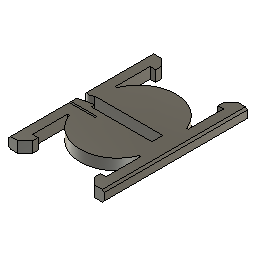
cable chain accessories v8 (Autodesk Fusion 360 design; units mm, degrees)
Autodesk Fusion 360 part; units mm, degrees
sketch "separator" plane through (0, 0, 0) normal (0, 0, 1) x (1, 0, 0)
  line L0 (0, 0) -> (57, 0)
  line L1 (57, 0) -> (57, 9)
  line L2 (57, 9) -> (0, 9)
  line L3 (0, 9) -> (0, 0)
  line L4 (0, 9) -> (57, 0) construction
  line L5 (41.5, 0) -> (15.5, 0) construction
  line L6 (15.5, 0) -> (15.5, 9)
  line L7 (15.5, 9) -> (41.5, 9) construction
  line L8 (41.5, 9) -> (41.5, 0)
  line L9 (41.5, 0) -> (15.5, 9) construction
  line L10 (15.5, 0) -> (41.5, 9) construction
  line L11 (12.5, 9) -> (12.5, 0)
  line L12 (44.5, 9) -> (44.5, 0)
  line L13 (16.5, 0) -> (16.5, 9)
  line L14 (40.5, 9) -> (40.5, 0)
  point P0 (28.5, 4.5)
  dimension "d1" = 57
  dimension "d2" = 9
  dimension "d3" = 26
  dimension "d4" = 9
  dimension "d5" = 3
  dimension "d6" = 3
  dimension "d7" = 1
  dimension "d8" = 1
  constraint horizontal L0
  constraint vertical L1
  constraint horizontal L2
  constraint vertical L3
  constraint coincident L0.start L3.end
  constraint horizontal L5
  constraint perpendicular L5 L6
  constraint parallel L5 L7
  constraint parallel L6 L8
  constraint coincident L9 P0
  constraint coincident L10 P0
  constraint midpoint L4 P0
  constraint coincident L2 L11.start
  constraint perpendicular L2 L11
  constraint coincident L2 L12.start
  constraint coincident L0 L12.end
  constraint perpendicular L0 L12
  measures "d1" distance of L0.start L0.end
  measures "d2" distance of L0.start L2.end
  measures "d3" distance of L6.end L7.end
  measures "d4" distance of L5.end L6.end
  measures "d5" distance of L6 L11
  measures "d6" distance of L8 L12
extrude "Extrude1" add sketch "separator" against normal blind 2 makes body 1
extrude "Extrude2" add sketch "separator" along normal blind 3.5 contours L0 L2 L6 L11 | L0 L2 L8 L12 bodies 1
extrude "Extrude3" add sketch "separator" along normal blind 1.5 from surface at 2 contours L0 L2 L6 L13 | L0 L2 L8 L14 bodies 1
fillet "Fillet1" radius 0.75 4 edges at (16.5, 4.5, 3.5) (16.5, 4.5, 2) (40.5, 4.5, 2) (40.5, 4.5, 3.5) on bodies 1
chamfer "Chamfer1" distance 1 angle 45 2 edges at (44.5, 4.5, 3.5) (12.5, 4.5, 3.5) on bodies 1
sketch "Sketch2" plane through (0, 0, 0) normal (0, 0, 1) x (1, 0, 0)
  line L0 (0, 0) -> (80, 0)
  line L1 (80, 0) -> (80, 39)
  line L2 (80, 39) -> (0, 39)
  line L3 (0, 39) -> (0, 0)
  line L4 (11, 39) -> (11, 0)
  line L5 (69, 39) -> (69, 0)
  line L6 (0, 6.5) -> (80, 6.5)
  line L7 (0, 39) -> (80, 0) construction
  line L8 (74.5, 11.5) -> (5.5, 11.5) construction
  line L9 (5.5, 11.5) -> (5.5, 27.5) construction
  line L10 (5.5, 27.5) -> (74.5, 27.5) construction
  line L11 (74.5, 27.5) -> (74.5, 11.5) construction
  line L12 (74.5, 11.5) -> (5.5, 27.5) construction
  line L13 (5.5, 11.5) -> (74.5, 27.5) construction
  circle A0 centre (5.5, 27.5) radius 2
  circle A1 centre (74.5, 27.5) radius 2
  circle A2 centre (5.5, 11.5) radius 2
  circle A3 centre (74.5, 11.5) radius 2
  arc A4 (13, 3) -> (22, 3) centre (17.5, 7.0625) ccw
  line L14 (22, 3) -> (22.6171, 6.5)
  line L15 (22, 3) -> (27, 3) construction
  line L16 (13, 3) -> (12.0622, 6.5)
  line L17 (13, 3) -> (16.8618, 3) construction
  line L18 (20.6035, 3.7181) -> (21.094, 6.5)
  arc A5 (14.3483, 3.7635) -> (20.6035, 3.7181) centre (17.5, 7.0625) ccw
  line L19 (14.3483, 3.7635) -> (13.6151, 6.5)
  arc A6 (24.5, 3) -> (33.5, 3) centre (29, 7.0625) ccw
  arc A7 (25.8483, 3.7635) -> (32.1035, 3.7181) centre (29, 7.0625) ccw
  line L20 (32.1035, 3.7181) -> (32.594, 6.5)
  line L21 (33.5, 3) -> (34.1171, 6.5)
  line L22 (25.8483, 3.7635) -> (25.1151, 6.5)
  line L23 (24.5, 3) -> (23.5622, 6.5)
  arc A8 (36, 3) -> (45, 3) centre (40.5, 7.0625) ccw
  arc A9 (37.3483, 3.7635) -> (43.6035, 3.7181) centre (40.5, 7.0625) ccw
  line L24 (43.6035, 3.7181) -> (44.094, 6.5)
  line L25 (45, 3) -> (45.6171, 6.5)
  line L26 (37.3483, 3.7635) -> (36.6151, 6.5)
  line L27 (36, 3) -> (35.0622, 6.5)
  arc A10 (47.5, 3) -> (56.5, 3) centre (52, 7.0625) ccw
  arc A11 (48.8483, 3.7635) -> (55.1035, 3.7181) centre (52, 7.0625) ccw
  line L28 (55.1035, 3.7181) -> (55.594, 6.5)
  line L29 (56.5, 3) -> (57.1171, 6.5)
  line L30 (48.8483, 3.7635) -> (48.1151, 6.5)
  line L31 (47.5, 3) -> (46.5622, 6.5)
  arc A12 (59, 3) -> (68, 3) centre (63.5, 7.0625) ccw
  arc A13 (60.3483, 3.7635) -> (66.6035, 3.7181) centre (63.5, 7.0625) ccw
  line L32 (66.6035, 3.7181) -> (67.094, 6.5)
  line L33 (68, 3) -> (68.6171, 6.5)
  line L34 (60.3483, 3.7635) -> (59.6151, 6.5)
  line L35 (59, 3) -> (58.0622, 6.5)
  point P0 (40, 19.5)
  dimension "d19" = 80
  dimension "d20" = 39
  dimension "d21" = 11
  dimension "d22" = 11
  dimension "d23" = 6.5
  dimension "d24" = 69
  dimension "d25" = 16
  dimension "d26" = 4
  dimension "d27" = 4
  dimension "d28" = 4
  dimension "d29" = 4
  dimension "d44" = 80
  dimension "d46" = 105
  dimension "d60" = 46
  dimension "d61" = 0
  constraint horizontal L0
  constraint vertical L1
  constraint horizontal L2
  constraint vertical L3
  constraint coincident L0.start L3.end
  constraint coincident L2 L4.start
  constraint coincident L0 L4.end
  constraint perpendicular L0 L4
  constraint coincident L2 L5.start
  constraint coincident L0 L5.end
  constraint perpendicular L0 L5
  constraint perpendicular L5 L6
  constraint horizontal L8
  constraint perpendicular L8 L9
  constraint parallel L8 L10
  constraint parallel L9 L11
  constraint coincident L12 P0
  constraint coincident L13 P0
  constraint midpoint L7 P0
  constraint coincident L9.end L10.start
  constraint coincident L10.end L11.start
  constraint coincident L8.end L9.start
  constraint coincident L8.start L11.end
  constraint coincident L3 L6.start
  constraint coincident L1 L6.end
  constraint horizontal L15
  constraint horizontal L17
  constraint coincident L6 L16.end
  constraint concentric A4 A5
  constraint coincident L6 L18.end
  constraint coincident L6 L14.end
  constraint coincident L6 L19.end
  measures "d19" distance of L0.start L0.end
  measures "d20" distance of L0.start L2.end
  measures "d21" distance of L3 L4
  measures "d22" distance of L1 L5
  measures "d23" distance of L0 L6
  measures "d24" distance of L9.end L10.end
  measures "d25" distance of L8.end L9.end
  measures "d26" diameter of A0
  measures "d27" diameter of A1
  measures "d28" diameter of A2
  measures "d29" diameter of A3
  measures "d44" angle of L14 L15
  measures "d46" angle of L16 L17
extrude "Extrude5" add sketch "Sketch2" along normal blind 40 separate body contours L0 L3 L4 L6 | L0 L4 L5 L6 A4 L14 L16 A6 L21 L23 A8 L25 L27 A10 L29 L31 A12 L33 L35 | L0 L1 L5 L6 | L6 A4 L14 L16 L18 A5 L19 | L6 A12 A13 L32 L33 L34 L35 | L6 L18 A5 L19 | L6 A13 L32 L34 | L6 A6 A7 L20 L21 L22 L23 | L6 A10 A11 L28 L29 L30 L31 | L6 A7 L20 L22 | L6 A11 L28 L30 | L6 A8 A9 L24 L25 L26 L27 | L6 A9 L24 L26 makes body 2
extrude "Extrude6" add sketch "Sketch2" along normal blind 25 contours L2 L3 L4 L6 | L1 L2 L5 L6 bodies 2
chamfer "Chamfer2" distance 15 angle 45 2 edges at (5.5, 39, 25) (74.5, 39, 25) on bodies 2
chamfer "Chamfer3" distance 5 angle 45 2 edges at (80, 3.25, 40) (0, 3.25, 40) on bodies 2
chamfer "Chamfer4" distance 1 angle 45 12 edges at (11, 15.25, 25) (11, 31.5, 17.5) (0, 31.5, 17.5) (0, 15.25, 25) (11, 39, 5) (0, 39, 5) (69, 39, 5) (80, 39, 5) (80, 31.5, 17.5) (69, 31.5, 17.5) (80, 15.25, 25) (69, 15.25, 25) on bodies 2
chamfer "Chamfer5" distance 1 angle 45 5 edges at (0, 6.5, 29.5) (2.5, 6.5, 37.5) (40, 6.5, 40) (77.5, 6.5, 37.5) (80, 6.5, 29.5) on bodies 2
extrude "Extrude10" cut sketch "Sketch2" along normal blind 3 from surface at 15 contours L6 A4 L14 L16 L18 A5 L19 | L6 A12 A13 L32 L33 L34 L35 | L6 A6 A7 L20 L21 L22 L23 | L6 A10 A11 L28 L29 L30 L31 | L6 A8 A9 L24 L25 L26 L27 bodies 2
extrude "Extrude11" cut sketch "Sketch2" along normal blind 3 from surface at 32 contours L6 A4 L14 L16 L18 A5 L19 | L6 A12 A13 L32 L33 L34 L35 | L6 A6 A7 L20 L21 L22 L23 | L6 A10 A11 L28 L29 L30 L31 | L6 A8 A9 L24 L25 L26 L27 bodies 2
chamfer "Chamfer6" distance 1 angle 45 5 edges at (80, 0, 17.5) (77.5, 0, 37.5) (40, 0, 40) (2.5, 0, 37.5) (0, 0, 17.5) on bodies 2
chamfer "Chamfer7" distance 1 angle 45 4 edges at (3.6353, 12.2232, 0) (3.6353, 28.2232, 0) (72.6353, 28.2232, 0) (72.6353, 12.2232, 0) on bodies 2
sketch "Sketch3" plane through (0, 0, 0) normal (0, 0, 1) x (1, 0, 0)
  line L0 (0, 0) -> (26, 0)
  line L1 (26, 0) -> (26, 39)
  line L2 (26, 39) -> (0, 39)
  line L3 (0, 39) -> (0, 0)
  line L4 (3, 35.5) -> (23, 35.5)
  line L5 (23, 35.5) -> (23, 32)
  line L6 (23, 32) -> (3, 32)
  line L7 (3, 32) -> (3, 35.5)
  line L8 (4.5, 39) -> (21.5, 39)
  line L9 (21.5, 39) -> (21.5, 35.5)
  line L10 (21.5, 35.5) -> (4.5, 35.5)
  line L11 (4.5, 35.5) -> (4.5, 39)
  line L12 (0, 19.5) -> (26, 19.5) construction
  line L13 (23, 7) -> (3, 7)
  line L14 (3, 7) -> (3, 3.5)
  line L15 (21.5, 3.5) -> (4.5, 3.5)
  line L16 (3, 3.5) -> (23, 3.5)
  line L17 (4.5, 3.5) -> (4.5, 0)
  line L18 (21.5, 0) -> (21.5, 3.5)
  line L19 (23, 3.5) -> (23, 7)
  line L20 (23, 7) -> (22.5, 7)
  line L21 (22.5, 7) -> (22.5, 13)
  line L22 (22.5, 13) -> (23, 13)
  line L23 (23, 13) -> (23, 7)
  line L24 (3, 7) -> (3.5, 7)
  line L25 (3.5, 7) -> (3.5, 13)
  line L26 (3.5, 13) -> (3, 13)
  line L27 (3, 13) -> (3, 7)
  line L28 (23, 32) -> (22.5, 32)
  line L29 (22.5, 32) -> (22.5, 26)
  line L30 (22.5, 26) -> (23, 26)
  line L31 (23, 26) -> (23, 32)
  line L32 (3, 32) -> (3.5, 32)
  line L33 (3.5, 32) -> (3.5, 26)
  line L34 (3.5, 26) -> (3, 26)
  line L35 (3, 26) -> (3, 32)
  arc A0 (22.5, 26) -> (3.5, 26) centre (13, 22.3563) ccw
  arc A1 (3.5, 13) -> (22.5, 13) centre (13, 16.6437) ccw
  dimension "d70" = 26
  dimension "d71" = 39
  dimension "d72" = 20
  dimension "d73" = 3.5
  dimension "d74" = 3
  dimension "d76" = 17
  dimension "d77" = 4.5
  dimension "d81" = 3.5
  dimension "d93" = 0.5
  dimension "d94" = 6
  dimension "d95" = 0.5
  dimension "d96" = 6
  dimension "d97" = 0.5
  dimension "d98" = 6
  dimension "d99" = 0.5
  dimension "d100" = 6
  constraint horizontal L0
  constraint vertical L1
  constraint horizontal L2
  constraint vertical L3
  constraint coincident L0.start L3.end
  constraint perpendicular L4 L5
  constraint parallel L4 L6
  constraint parallel L5 L7
  constraint perpendicular L1 L4
  constraint horizontal L8
  constraint vertical L9
  constraint horizontal L10
  constraint vertical L11
  constraint coincident L4 L9.end
  constraint coincident L2 L8.start
  constraint midpoint L3 L12.start
  constraint midpoint L1 L12.end
  constraint symmetric L4.start L12 L14.end
  constraint symmetric L4.end L12 L16.end
  constraint symmetric L5.end L12 L13.start
  constraint symmetric L6.end L12 L13.end
  constraint symmetric L8.start L12 L17.end
  constraint symmetric L8.end L12 L18.start
  constraint symmetric L9.end L12 L15.start
  constraint symmetric L10.end L12 L15.end
  constraint horizontal L20
  constraint vertical L21
  constraint horizontal L22
  constraint vertical L23
  constraint horizontal L24
  constraint vertical L25
  constraint horizontal L26
  constraint vertical L27
  constraint horizontal L28
  constraint vertical L29
  constraint horizontal L30
  constraint vertical L31
  constraint horizontal L32
  constraint vertical L33
  constraint horizontal L34
  constraint vertical L35
  constraint symmetric L12 L29.end L21.end
  constraint symmetric L12 L33.end L25.end
  constraint symmetric L12 A0 A1
  measures "d70" distance of L0.start L0.end
  measures "d71" distance of L0.start L2.end
  measures "d72" distance of L4.start L4.end
  measures "d73" distance of L4.start L6.end
  measures "d74" distance of L3 L7
  measures "d76" distance of L8.start L8.end
  measures "d77" distance of L3 L11
  measures "d81" distance of L2 L4
  measures "d93" distance of L13.start L20.end
  measures "d94" distance of L13.start L22.end
  measures "d95" distance of L13.end L24.end
  measures "d96" distance of L13.end L26.end
  measures "d97" distance of L5.end L28.end
  measures "d98" distance of L5.end L30.end
  measures "d99" distance of L6.end L32.end
  measures "d100" distance of L6.end L34.end
extrude "Extrude12" add sketch "Sketch3" along normal blind 3 separate body contours L0 L1 L2 L3 L4 L5 L6 L7 L9 L11 L13 L14 L16 L17 L18 L19 L22 L23 L26 L27 L30 L31 L34 L35 A0 A1 | L13 L24 L25 L26 L27 | L13 L20 L21 L22 L23 | L13 L25 A1 | L6 L32 L33 L34 L35 | L13 L21 A1 | L6 L28 L29 L30 L31 | L6 L33 A0 | L6 L29 A0 makes body 3
sketch "Sketch4" plane through (0, 0, 0) normal (0, 0, -1) x (1, 0, 0)
  line L0 (0, 0) -> (0, -39)
  line L1 (0, -39) -> (4.5, -39)
  line L2 (4.5, -39) -> (4.5, -35.5)
  line L3 (4.5, -35.5) -> (3, -35.5)
  line L4 (3, -35.5) -> (3, -32)
  line L5 (3, -32) -> (23, -32)
  line L6 (23, -32) -> (23, -35.5)
  line L7 (23, -35.5) -> (21.5, -35.5)
  line L8 (21.5, -35.5) -> (21.5, -39)
  line L9 (21.5, -39) -> (26, -39)
  line L10 (26, -39) -> (26, 0)
  line L11 (26, 0) -> (21.5, 0)
  line L12 (21.5, 0) -> (21.5, -3.5)
  line L13 (21.5, -3.5) -> (23, -3.5)
  line L14 (23, -3.5) -> (23, -7)
  line L15 (23, -7) -> (3, -7)
  line L16 (3, -7) -> (3, -3.5)
  line L17 (3, -3.5) -> (4.5, -3.5)
  line L18 (4.5, -3.5) -> (4.5, 0)
  line L19 (4.5, 0) -> (0, 0)
  line L20 (23, -32) -> (3, -7) construction
  line L21 (21, -18) -> (5, -18)
  line L22 (5, -18) -> (5, -21)
  line L23 (5, -21) -> (21, -21)
  line L24 (21, -21) -> (21, -18)
  line L25 (21, -18) -> (5, -21) construction
  line L26 (5, -18) -> (21, -21) construction
  line L27 (5, -21) -> (0, -21)
  line L28 (5, -18) -> (0, -18)
  line L29 (4.5, -19) -> (0, -18)
  line L30 (4.5, -19) -> (4.5, -18)
  line L31 (0, -16.5) -> (7.5, -16.5)
  line L32 (7.5, -16.5) -> (7.5, -16)
  line L33 (7.5, -16) -> (0, -16)
  line L34 (0, -16) -> (0, -16.5)
  arc A0 (2.5, -21) -> (0, -21) centre (1.25, -22.31) ccw
  point P0 (13, -19.5)
  dimension "d89" = 16
  dimension "d90" = 3
  constraint coincident L5.end L6.start
  constraint coincident L15.end L16.start
  constraint horizontal L21
  constraint perpendicular L21 L22
  constraint parallel L21 L23
  constraint parallel L22 L24
  constraint coincident L25 P0
  constraint coincident L26 P0
  constraint midpoint L20 P0
  constraint perpendicular L22 L27
  constraint coincident L0 L28.end
  constraint perpendicular L0 L28
  constraint coincident L28 L30.end
  constraint perpendicular L28 L30
  constraint horizontal L31
  constraint vertical L32
  constraint horizontal L33
  constraint vertical L34
  constraint coincident L0 L31.start
  constraint midpoint L27 A0.start
  measures "d89" distance of L22.end L23.end
  measures "d90" distance of L21.end L22.end
extrude "Extrude14" cut sketch "Sketch4" against normal blind 3 contours L0 L31 L32 L33 L34 | L0 L22 L27 L28 L29 L30 A0 | L27 A0 | L21 L22 L23 L24 bodies 3
extrude "Extrude15" cut sketch "Sketch3" along normal blind 3 contours L13 L24 L25 L26 L27 | L13 L20 L21 L22 L23 | L6 L32 L33 L34 L35 | L6 L28 L29 L30 L31 bodies 3
sketch "Sketch5" plane through (0, 0, 0) normal (0, 0, -1) x (1, 0, 0)
  line L0 (3.5, -26) -> (3.5, -32)
  line L1 (3.5, -32) -> (22.5, -32)
  line L2 (22.5, -32) -> (22.5, -26)
  line L3 (22.5, -26) -> (23, -26)
  line L4 (23, -26) -> (23, -35.5)
  line L5 (23, -35.5) -> (21.5, -35.5)
  line L6 (21.5, -35.5) -> (21.5, -39)
  line L7 (21.5, -39) -> (26, -39)
  line L8 (26, -39) -> (26, 0)
  line L9 (26, 0) -> (21.5, 0)
  line L10 (21.5, 0) -> (21.5, -3.5)
  line L11 (21.5, -3.5) -> (23, -3.5)
  line L12 (23, -3.5) -> (23, -13)
  line L13 (23, -13) -> (22.5, -13)
  line L14 (22.5, -13) -> (22.5, -7)
  line L15 (22.5, -7) -> (3.5, -7)
  line L16 (3.5, -7) -> (3.5, -13)
  line L17 (3.5, -13) -> (3, -13)
  line L18 (3, -13) -> (3, -3.5)
  line L19 (3, -3.5) -> (4.5, -3.5)
  line L20 (4.5, -3.5) -> (4.5, 0)
  line L21 (4.5, 0) -> (0, 0)
  line L22 (0, 0) -> (0, -16)
  line L23 (0, -16) -> (7.5, -16)
  line L24 (7.5, -16) -> (7.5, -16.5)
  line L25 (7.5, -16.5) -> (0, -16.5)
  line L26 (0, -16.5) -> (0, -18)
  line L27 (0, -18) -> (4.5, -19)
  line L28 (4.5, -19) -> (4.5, -18)
  line L29 (4.5, -18) -> (21, -18)
  line L30 (21, -18) -> (21, -21)
  line L31 (21, -21) -> (0, -21)
  line L32 (0, -39) -> (4.5, -39)
  line L33 (4.5, -39) -> (4.5, -35.5)
  line L34 (4.5, -35.5) -> (3, -35.5)
  line L35 (3, -35.5) -> (3, -26)
  line L36 (3, -26) -> (3.5, -26)
  line L37 (27, -21) -> (-1, -21)
  line L38 (-1, -21) -> (-1, -18)
  line L39 (-1, -18) -> (27, -18)
  line L40 (27, -18) -> (27, -21)
  line L41 (0, -21) -> (0, -18)
  line L42 (4.5, -19) -> (4.5, -21)
  line L43 (20.5, -21) -> (20.5, -18)
  line L44 (5, -21) -> (5, -18)
  line L45 (0, -21) -> (0, -39)
  dimension "d113" = 0.5
  dimension "d114" = 0.5
  constraint horizontal L37
  constraint vertical L38
  constraint horizontal L39
  constraint vertical L40
  constraint coincident L31.end L41.start
  constraint coincident L26.end L27.start
  constraint coincident L27.end L28.start
  constraint coincident L37 L42.end
  constraint perpendicular L37 L42
  constraint coincident L31 L43.start
  constraint coincident L29 L43.end
  constraint perpendicular L29 L43
  constraint coincident L31 L44.start
  constraint coincident L39 L44.end
  constraint perpendicular L39 L44
  measures "d113" distance of L30 L43
  measures "d114" distance of L42 L44
extrude "Extrude16" add sketch "Sketch5" along normal blind 57 separate body contours L27 L31 L37 L41 L42 | L28 L29 L31 L37 L39 L42 L44 | L27 L28 L39 | L29 L31 L37 L39 L43 L44 | L8 L30 L37 L39 | L29 L30 L31 L37 L39 L43 makes body 4
extrude "Extrude17" cut sketch "Sketch5" along normal blind 3 from surface at 10 contours L27 L31 L37 L41 L42 | L28 L29 L31 L37 L39 L42 L44 | L27 L28 L39 | L8 L30 L37 L39 | L29 L30 L31 L37 L39 L43 bodies 4
extrude "Extrude18" cut sketch "Sketch5" along normal blind 3 from surface at 29 contours L27 L31 L37 L41 L42 | L28 L29 L31 L37 L39 L42 L44 | L27 L28 L39 | L8 L30 L37 L39 | L29 L30 L31 L37 L39 L43 bodies 4
chamfer "Chamfer9" distance 0.5 angle 45 12 edges at (26, 18, -44.5) (26, 18, -21) (26, 18, -5) (0, 18, -5) (0, 18, -21) (0, 18, -44.5) (0, 21, -44.5) (0, 21, -21) (0, 21, -5) (26, 21, -44.5) (26, 21, -21) (26, 21, -5) on bodies 4
extrude "Extrude19" add sketch "Sketch4" against normal blind 3 contours L27 A0 bodies 3
chamfer "Chamfer10" distance 0.5 angle 45 12 edges at (26, 19.5, 3) (26, 19.5, 0) (0, 17.25, 0) (0, 30, 0) (0, 8, 0) (0, 17.25, 3) (0, 8, 3) (0, 30, 3) (0, 8, 0) (0, 8, 3) (0, 17.25, 0) (0, 17.25, 3) on bodies 3
chamfer "Chamfer11" distance 2 angle 45 4 edges at (4.5, 0, 1.5) (21.5, 0, 1.5) (4.5, 39, 1.5) (21.5, 39, 1.5) on bodies 3
chamfer "Chamfer12" distance 3 angle 45 4 edges at (3.5, 7, 1.5) (22.5, 7, 1.5) (22.5, 32, 1.5) (3.5, 32, 1.5) on bodies 3
extrude "Extrude20" cut sketch "Sketch3" along normal blind 3 contours L6 L33 A0 | L6 L29 A0 bodies 3
extrude "Extrude21" add sketch "Sketch3" along normal blind 3 contours L6 A0 bodies 3
extrude "Extrude22" add sketch "Sketch3" along normal blind 3 contours L13 A1 bodies 3
extrude "Extrude23" cut sketch "Sketch3" along normal blind 3 contours L13 L25 A1 | L13 L21 A1 bodies 3
extrude "Extrude13" [suppressed]
hidden bodies 1 2 4
